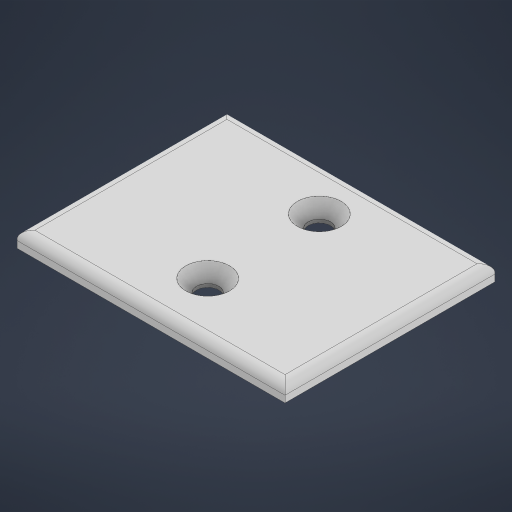
# Autodesk Inventor part: ShortSideMount
Saved by Autodesk Inventor 2024 (Build 280153000, 153)
## iProperties
Created: 2024-02-05
Part Number: ShortSideMount
Material: Generic
Document SubType Name: Modeling
Designer: Decla
Density: 1 g/cm^3
Appearance: Default
Author: Decla
Autodesk Inventor part; units mm, degrees
ref_plane "YZ Plane" through (0, 0, 0) normal (1, 0, 0) x (0, 1, 0)
ref_plane "XZ Plane" through (0, 0, 0) normal (0, 1, 0) x (-1, 0, 0)
ref_plane "XY Plane" through (0, 0, 0) normal (0, 0, 1) x (1, 0, 0)
sketch "Sketch1" plane through (0, 0, 0) normal (0, 1, 0) x (-1, 0, 0)
  line L0 (0, 0) -> (-60, 0)
  line L1 (-60, 0) -> (-60, -47)
  line L2 (-60, -47) -> (0, -47)
  line L3 (0, -47) -> (0, 0)
  point P0 (-30, -47)
  point P1 (-30, 0)
  dimension "d0" = 60
  dimension "d1" = 47
  constraints: 8 end point, 2 midpoint, 2 parallel, 1 horizontal, 1 perpendicular
  measures "d0" distance of L2.end L1.end
  measures "d1" distance of L1.end L0.end
extrude "Extrusion1" add sketch "Sketch1" along normal blind 3.5
sketch "Sketch2" plane through (0, 3.5, 0) normal (0, 1, 0) x (1, 0, 0)
  line L0 (0, 0) -> (60, 0) projected
  line L1 (60, 47) -> (0, 47) projected
  point P0 (30.6818, 37)
  point P1 (30.6818, 12)
  point P2 (30, 0)
  dimension "d10" = 25
  dimension "d11" = 12
  dimension "d12" = 10
  constraints: 1 midpoint
  measures "d10" distance of point (30.682, 12) point (30.682, 37)
  measures "d11" vertical distance of point (30, 0) point (30.682, 12)
  measures "d12" distance from line of L1 point (30.682, 37)
hole "Hole1" at (30.6818, 3.5, -37) at (30.6818, 3.5, -12) direction (0, -1, 0) diameter 4.978 end through all countersink diameter 9.779 countersink angle 82 clearance for "Flat Head Machine Screw (82)" size "#10" standard "Ansi Unified Screw Threads"
fillet "Fillet2" radius 2 4 edges at (30, 3.5, -47) (0, 3.5, -23.5) (30, 3.5, 0) (60, 3.5, -23.5) curvature continuous yes
body "Solid1"
